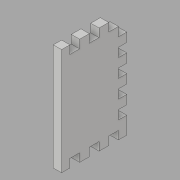
# Autodesk Inventor part: g_arm_v_3
Saved by Autodesk Inventor 2019 (Build 230136000, 136)
## iProperties
Created: 2021-11-02
Part Number: g_arm_v_3
Material: Generic
Document SubType Name: Modeling
Designer: Mohamed
Density: 1 g/cm^3
Appearance: Default
Author: Mohamed
Autodesk Inventor part; units mm, degrees
ref_plane "YZ Plane" through (0, 0, 0) normal (1, 0, 0) x (0, 1, 0)
ref_plane "XZ Plane" through (0, 0, 0) normal (0, 1, 0) x (-1, 0, 0)
ref_plane "XY Plane" through (0, 0, 0) normal (0, 0, 1) x (1, 0, 0)
sketch "Sketch1" plane through (0, 0, 0) normal (1, 0, 0) x (0, 1, 0)
  line L0 (0, 0) -> (77, 0)
  line L1 (77, 0) -> (77, -47)
  line L2 (77, -47) -> (0, -47)
  line L3 (0, -47) -> (0, 0)
  dimension "d0" = 77
  dimension "d1" = 47
  constraints: 8 end point, 2 parallel, 1 horizontal, 1 perpendicular
  measures "d0" distance of L1.end L2.end
  measures "d1" distance of L0.end L1.end
extrude "Extrusion1" add sketch "Sketch1" along normal blind 6
sketch "Sketch2" plane through (6, 0, 0) normal (1, 0, 0) x (0, 0, -1)
  line L0 (47, 0) -> (47, 77) projected
  line L1 (47, 77) -> (47, 71)
  line L2 (47, 71) -> (41, 71)
  line L3 (41, 71) -> (41, 64.5)
  line L4 (41, 64.5) -> (47, 64.5)
  line L5 (47, 64.5) -> (47, 71)
  point P0 (0, 0)
  dimension "d4" = 6
  dimension "d5" = 6
  dimension "d6" = 6.5
  constraints: 10 end point, 2 parallel, 1 horizontal, 1 perpendicular, 1 point on line
  measures "d4" distance of L0.end L1.end
  measures "d5" distance of L4.end L3.end
  measures "d6" distance of L3.end L2.end
extrude "Extrusion2" cut sketch "Sketch2" against normal blind 6
pattern_linear "Rectangular Pattern1" count 5 spacing 13 along (0, -1, 0) of "Extrusion2"
sketch "Sketch3" plane through (6, 0, 0) normal (1, 0, 0) x (0, 0, -1)
  line L0 (0, 77) -> (0, 0) projected
  line L1 (0, 77) -> (6, 77)
  line L2 (47, 77) -> (0, 77) projected
  line L3 (6, 77) -> (13, 77)
  line L4 (13, 77) -> (13, 71)
  line L5 (13, 71) -> (6, 71)
  line L6 (6, 71) -> (6, 77)
  line L7 (0, 0) -> (47, 0) projected
  line L8 (0, 0) -> (6, 0)
  line L9 (6, 0) -> (13, 0)
  line L10 (13, 0) -> (13, 6)
  line L11 (13, 6) -> (6, 6)
  line L12 (6, 6) -> (6, 0)
  dimension "d12" = 6
  dimension "d13" = 7
  dimension "d14" = 6
  dimension "d15" = 6
  dimension "d16" = 7
  dimension "d17" = 6
  constraints: 20 end point, 4 parallel, 2 horizontal, 2 perpendicular, 2 point on line
  measures "d12" distance of L0.start L1.end
  measures "d13" distance of L4.end L5.end
  measures "d14" distance of L3.end L4.end
  measures "d15" distance of L0.end L8.end
  measures "d16" distance of L11.end L10.end
  measures "d17" distance of L10.end L9.end
extrude "Extrusion3" cut sketch "Sketch3" against normal blind 6
pattern_linear "Rectangular Pattern2" count 3 spacing 14 along (0, 0, -1) of "Extrusion3"
sketch "Sketch4" plane through (6, 0, 0) normal (1, 0, 0) x (0, 0, -1)
  line L0 (47, 76.8975) -> (47, 71)
  line L1 (41, 71) -> (47, 71) projected
  line L2 (47, 71) -> (47, 77) projected
  line L3 (41, 71) -> (47, 71)
  line L4 (47, 71) -> (47, 77)
  line L5 (47, 77) -> (41, 77)
  line L6 (41, 77) -> (41, 71)
  point P0 (0, 0)
  constraints: 10 end point, 2 parallel, 1 horizontal, 1 perpendicular
extrude "Extrusion4" cut sketch "Sketch4" against normal blind 6
body "Solid1"
